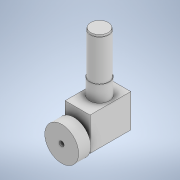
# Autodesk Inventor part: Bloc-moteur
Saved by Autodesk Inventor 2020 (Build 240168000, 168)
## iProperties
Created: 2019-11-28
Part Number: Bloc-moteur
Material: Générique
Document SubType Name: Modeling
Designer: change_le_nom
Density: 1 g/cm^3
Appearance: Par défaut
Author: change_le_nom
Autodesk Inventor part; units mm, degrees
ref_plane "YZ Plane" through (0, 0, 0) normal (1, 0, 0) x (0, 1, 0)
ref_plane "XZ Plane" through (0, 0, 0) normal (0, 1, 0) x (-1, 0, 0)
ref_plane "XY Plane" through (0, 0, 0) normal (0, 0, 1) x (1, 0, 0)
sketch "Esquisse1" plane through (0, 0, 0) normal (0, 1, 0) x (-1, 0, 0)
  line L0 (0, 0) -> (40.2, 0)
  line L1 (40.2, 0) -> (40.2, -65.7)
  line L2 (40.2, -65.7) -> (0, -65.7)
  line L3 (0, -65.7) -> (0, 0)
  dimension "d2" = 40.2
  dimension "d3" = 65.7
  constraints: 8 end point, 2 parallel, 1 horizontal, 1 perpendicular
  measures "d2" distance of L1.end L2.end
  measures "d3" distance of L0.end L1.end
extrude "Extrusion1" add sketch "Esquisse1" along normal blind 10.2
sketch "Esquisse2" plane through (-40.2, 0, 0) normal (0, 0, 1) x (1, 0, 0)
  line L0 (0, 0) -> (40.2, 0)
  line L1 (40.2, 0) -> (40.2, -43.4)
  line L2 (40.2, -43.4) -> (0, -43.4)
  line L3 (0, -43.4) -> (0, 0)
  dimension "d6" = 43.4
  constraints: 8 end point, 2 parallel, 1 horizontal, 1 perpendicular
  measures "d6" distance of L0.end L1.end
extrude "Extrusion2" add sketch "Esquisse2" against normal blind 12
sketch "Esquisse3" plane through (0, 10.2, 0) normal (0, 1, 0) x (1, 0, 0)
  line L0 (-40.2, 0) -> (0, 0) projected
  line L1 (0, 65.7) -> (-40.2, 65.7) projected
  line L2 (0, 12) -> (0, 65.7) projected
  line L3 (-40.2, 65.7) -> (0, 65.7)
  line L4 (0, 65.7) -> (0, 51.5)
  line L5 (0, 51.5) -> (-40.2, 51.5)
  line L6 (-40.2, 51.5) -> (-40.2, 65.7)
  line L7 (0, 0) -> (0, 65.7) projected
  line L8 (-40.2, 0) -> (0, 0)
  line L9 (0, 0) -> (0, 19.2)
  line L10 (0, 19.2) -> (-40.2, 19.2)
  line L11 (-40.2, 19.2) -> (-40.2, 0)
  circle A0 centre (-20.1, 35.35) radius 15.825
  dimension "d9" = 14.2
  dimension "d10" = 19.2
  dimension "d12" = 31.65
  constraints: 16 end point, 4 parallel, 2 horizontal, 2 perpendicular, 2 point on line, 1 centre point
  measures "d9" distance of L3.end L4.end
  measures "d10" distance of L9.end L8.end
  measures "d12" diameter of A0
extrude "Extrusion3" add sketch "Esquisse3" along normal blind 26.2 contours A0
sketch "Esquisse4" plane through (-20.1, 36.4, -35.35) normal (0, 1, 0) x (1, 0, 0)
  circle A0 centre (0, 0) radius 15
  point P0 (20.1, -35.35)
  dimension "d15" = 30
  constraints: 1 centre point
  measures "d15" diameter of A0
extrude "Extrusion4" add sketch "Esquisse4" along normal blind 65.35
sketch "Esquisse5" plane through (-20.1, 101.75, -35.35) normal (0, 1, 0) x (1, 0, 0)
  circle A0 centre (0, 0) radius 14.1
  point P0 (20.1, -35.35)
  dimension "d18" = 28.2
  constraints: 1 centre point
  measures "d18" diameter of A0
extrude "Extrusion5" add sketch "Esquisse5" along normal blind 3
sketch "Esquisse6" plane through (-40.2, 10.2, 0) normal (0, 0, 1) x (1, 0, 0)
  line L0 (0, -53.6) -> (40.2, -53.6) projected
  line L1 (0, -53.6) -> (16.2, -53.6)
  line L2 (0, -37.4) -> (0, -53.6)
  line L3 (40.2, -53.6) -> (40.2, 0) projected
  line L4 (40.2, -53.6) -> (24, -53.6)
  line L5 (40.2, -37.4) -> (40.2, -53.6)
  circle A0 centre (20.1, -37.4) radius 4
  point P0 (40.2, -10.2)
  dimension "d25" = 8
  constraints: 8 end point, 2 horizontal, 1 centre point
  measures "d25" diameter of A0
extrude "Extrusion6" add sketch "Esquisse6" along normal blind 6
sketch "Esquisse7" plane through (-20.1, -27.2, 6) normal (0, 0, 1) x (1, 0, 0)
  circle A0 centre (0, 0) radius 4 projected
  circle A1 centre (0, 0) radius 27.3
  point P0 (20.1, 27.2)
  dimension "d28" = 54.6
  constraints: 1 centre point, 1 coincident
  measures "d28" diameter of A1
extrude "Extrusion7" add sketch "Esquisse7" along normal blind 19.6
sketch "Esquisse8" plane through (0, 0, -65.7) normal (1, 0, 0) x (0, 0, -1)
  line L0 (-53.7, 0) -> (0, 0) projected
  line L1 (-53.7, 0) -> (-53.7, -43.4) projected
  line L2 (0, 0) -> (-53.7, 0)
  line L3 (-53.7, 0) -> (-53.7, -43.4)
  line L4 (-53.7, -43.4) -> (0, -43.4)
  line L5 (0, -43.4) -> (0, 0)
  point P0 (-65.7, 0)
  constraints: 8 end point, 2 parallel, 1 horizontal, 1 perpendicular
extrude "Extrusion8" add sketch "Esquisse8" against normal blind 40.2
